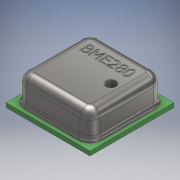
# Autodesk Inventor part: 66-0007
Saved by Autodesk Inventor 2018 (Build 220112000, 112)
## iProperties
Created: 2020-01-30
Part Number: 66-0007
Material: Stainless Steel
Document SubType Name: Modeling
Designer: Bradley
Density: 8 g/cm^3
Appearance: Semi-Polished
Author: Bradley
Autodesk Inventor part; units mm, degrees
ref_plane "YZ Plane" through (0, 0, 0) normal (1, 0, 0) x (0, 1, 0)
ref_plane "XZ Plane" through (0, 0, 0) normal (0, 1, 0) x (-1, 0, 0)
ref_plane "XY Plane" through (0, 0, 0) normal (0, 0, 1) x (1, 0, 0)
sketch "Sketch1" plane through (0, 0, 0) normal (0, 0, 1) x (1, 0, 0)
  line L0 (-1.25, 1.25) -> (1.25, 1.25)
  line L1 (1.25, 1.25) -> (1.25, -1.25)
  line L2 (1.25, -1.25) -> (-1.25, -1.25)
  line L3 (-1.25, -1.25) -> (-1.25, 1.25)
  line L4 (-1.25, 1.25) -> (1.25, -1.25) construction
  line L5 (1.25, 1.25) -> (-1.25, -1.25) construction
  point P0 (0, 0)
  dimension "d0" = 2.5
  constraints: 12 end point, 2 midpoint, 2 parallel, 2 perpendicular, 1 horizontal
  measures "d0" distance of L1.end L2.end
extrude "Extrusion1" add sketch "Sketch1" along normal mid plane 0.13
sketch "Sketch2" plane through (0, 0, 0.065) normal (0, 0, 1) x (1, 0, 0)
  line L0 (1.25, 1.25) -> (-1.25, 1.25) projected
  line L1 (-1.25, 1.25) -> (-1.25, -1.25) projected
  line L2 (-1.25, -1.25) -> (1.25, -1.25) projected
  line L3 (1.25, -1.25) -> (1.25, 1.25) projected
  line L4 (-1.1, 1.1) -> (1.1, 1.1)
  line L5 (1.1, 1.1) -> (1.1, -1.1)
  line L6 (1.1, -1.1) -> (-1.1, -1.1)
  line L7 (-1.1, -1.1) -> (-1.1, 1.1)
  point P0 (0, 0)
  dimension "d3" = 2.2
  constraints: 8 end point, 3 other
  measures "d3" distance of L4.start L4.end
extrude "Extrusion2" add sketch "Sketch2" along normal blind 0.8 contours L4 L5 L6 L7
fillet "Fillet1" radius 0.3 4 edges at (1.1, 1.1, 0.465) (-1.1, 1.1, 0.465) (-1.1, -1.1, 0.465) (1.1, -1.1, 0.465)
fillet "Fillet1" radius 0.25 4 edges at (0, 1.1, 0.865) (-1.1, 0, 0.865) (1.1, 0, 0.865) (0, -1.1, 0.865)
fillet "Fillet1" radius 0.15 4 edges at (0, -1.1, 0.065) (1.1, 0, 0.065) (0, 1.1, 0.065) (-1.1, 0, 0.065)
sketch "Sketch3" plane through (0, 0, 0.865) normal (0, 0, 1) x (1, 0, 0)
  arc A0 (0.85, 0.8) -> (0.8, 0.85) centre (0.8, 0.8) ccw projected
  line L0 (-0.8, 0.85) -> (0.8, 0.85) projected
  arc A1 (-0.8, 0.85) -> (-0.85, 0.8) centre (-0.8, 0.8) ccw projected
  line L1 (-0.85, -0.8) -> (-0.85, 0.8) projected
  arc A2 (-0.85, -0.8) -> (-0.8, -0.85) centre (-0.8, -0.8) ccw projected
  line L2 (0.8, -0.85) -> (-0.8, -0.85) projected
  arc A3 (0.8, -0.85) -> (0.85, -0.8) centre (0.8, -0.8) ccw projected
  line L3 (0.85, 0.8) -> (0.85, -0.8) projected
  arc A4 (1.15, 0.8) -> (0.8, 1.15) centre (0.8, 0.8) ccw
  line L4 (1.15, 0.8) -> (1.15, -0.8)
  arc A5 (0.8, -1.15) -> (1.15, -0.8) centre (0.8, -0.8) ccw
  line L5 (0.8, -1.15) -> (-0.8, -1.15)
  arc A6 (-1.15, -0.8) -> (-0.8, -1.15) centre (-0.8, -0.8) ccw
  line L6 (-1.15, -0.8) -> (-1.15, 0.8)
  arc A7 (-0.8, 1.15) -> (-1.15, 0.8) centre (-0.8, 0.8) ccw
  line L7 (-0.8, 1.15) -> (0.8, 1.15)
  line L8 (-1.25, 1.25) -> (1.25, 1.25) projected
  line L9 (1.25, 1.25) -> (1.25, -1.25) projected
  line L10 (1.25, -1.25) -> (-1.25, -1.25) projected
  line L11 (-1.25, -1.25) -> (-1.25, 1.25) projected
  point P0 (0, 0)
  dimension "d9" = 2.3
  constraints: 8 end point, 8 point on circle, 4 centre point, 7 other
  measures "d9" distance between parallel lines of L4 L6
extrude "Extrusion3" cut sketch "Sketch3" against normal up to surface (0.8 mm away) contours L8 L9 L10 L11
sketch "Sketch4" plane through (0, 0, 0.865) normal (0, 0, 1) x (1, 0, 0)
  circle A0 centre (0.625, 0) radius 0.15
  line L0 (1.25, -1.25) -> (1.25, 1.25) projected
  point P0 (0, 0)
  dimension "d12" = 0.3
  dimension "d13" = 0.625
  constraints: 1 centre point, 1 horizontal alignment
  measures "d12" diameter of A0
  measures "d13" distance from line of L0 A0.centre
extrude "Extrusion4" cut sketch "Sketch4" against normal blind 0.8
sketch "Sketch5" plane through (0, 0, -0.065) normal (0, 0, -1) x (-1, 0, 0)
  line L0 (1.25, 1.25) -> (-1.25, 1.25) projected
  line L1 (-1.25, 1.25) -> (-1.25, -1.25) projected
  line L2 (-1.25, -1.25) -> (1.25, -1.25) projected
  line L3 (1.25, -1.25) -> (1.25, 1.25) projected
  line L4 (1.15, 1.15) -> (0.8, 1.15)
  line L5 (0.8, 1.15) -> (0.8, 0.8)
  line L6 (0.8, 0.8) -> (1.15, 0.8)
  line L7 (1.15, 0.8) -> (1.15, 1.15)
  line L8 (-1.15, 1.15) -> (-1.15, 0.8)
  line L9 (-1.15, 0.8) -> (-0.8, 0.8)
  line L10 (-0.8, 0.8) -> (-0.8, 1.15)
  line L11 (-0.8, 1.15) -> (-1.15, 1.15)
  line L12 (0.8, 0.5) -> (0.8, 0.15)
  line L13 (0.8, 0.15) -> (1.15, 0.15)
  line L14 (1.15, 0.15) -> (1.15, 0.5)
  line L15 (1.15, 0.5) -> (0.8, 0.5)
  line L16 (-1.15, 0.5) -> (-1.15, 0.15)
  line L17 (-1.15, 0.15) -> (-0.8, 0.15)
  line L18 (-0.8, 0.15) -> (-0.8, 0.5)
  line L19 (-0.8, 0.5) -> (-1.15, 0.5)
  line L20 (0.8, -0.15) -> (0.8, -0.5)
  line L21 (0.8, -0.5) -> (1.15, -0.5)
  line L22 (1.15, -0.5) -> (1.15, -0.15)
  line L23 (1.15, -0.15) -> (0.8, -0.15)
  line L24 (-1.15, -0.15) -> (-1.15, -0.5)
  line L25 (-1.15, -0.5) -> (-0.8, -0.5)
  line L26 (-0.8, -0.5) -> (-0.8, -0.15)
  line L27 (-0.8, -0.15) -> (-1.15, -0.15)
  line L28 (0.8, -0.8) -> (0.8, -1.15)
  line L29 (0.8, -1.15) -> (1.15, -1.15)
  line L30 (1.15, -1.15) -> (1.15, -0.8)
  line L31 (1.15, -0.8) -> (0.8, -0.8)
  line L32 (-1.15, -0.8) -> (-1.15, -1.15)
  line L33 (-1.15, -1.15) -> (-0.8, -1.15)
  line L34 (-0.8, -1.15) -> (-0.8, -0.8)
  line L35 (-0.8, -0.8) -> (-1.15, -0.8)
  circle A0 centre (-0.5, -0.975) radius 0.1
  point P0 (0, 0)
  point P1 (-0.8, -0.975)
  dimension "d16" = 0.35
  dimension "d19" = 1.95
  dimension "d22" = 0.65
  dimension "d25" = 0.75
  dimension "d26" = 0.1
  dimension "d27" = 0.1
  dimension "d28" = 0.2
  constraints: 64 end point, 2 horizontal, 2 parallel, 2 perpendicular, 1 centre point, 1 horizontal alignment, 1 midpoint, 1 vertical, 56 other
  measures "d16" distance of L6.end L5.end
  measures "d19" distance of L4.end L8.start
  measures "d22" distance of L4.end L12.start
  measures "d25" distance from line of A0.centre L1
  measures "d26" distance between parallel lines of L2 L29
  measures "d27" distance between parallel lines of L3 L30
  measures "d28" diameter of A0
extrude "Extrusion5" add sketch "Sketch5" along normal blind 0.02 contours L7 L6 L5 L4 | L11 L10 L9 L8 | L15 L14 L13 L12 | L19 L18 L17 L16 | L23 L22 L21 L20 | L27 L26 L25 L24 | L31 L30 L29 L28 | L35 L34 L33 L32 | A0
sketch "Sketch6" plane through (0, 0, 0.865) normal (0, 0, 1) x (1, 0, 0)
  circle A0 centre (0.625, 0) radius 0.15 construction
  arc A1 (0.85, 0.8) -> (0.8, 0.85) centre (0.8, 0.8) ccw construction
  line L0 (-0.8, 0.85) -> (0.8, 0.85) construction
  arc A2 (-0.8, 0.85) -> (-0.85, 0.8) centre (-0.8, 0.8) ccw construction
  line L1 (-0.85, -0.8) -> (-0.85, 0.8) construction
  arc A3 (-0.85, -0.8) -> (-0.8, -0.85) centre (-0.8, -0.8) ccw construction
  line L2 (0.8, -0.85) -> (-0.8, -0.85) construction
  arc A4 (0.8, -0.85) -> (0.85, -0.8) centre (0.8, -0.8) ccw construction
  line L3 (0.85, 0.8) -> (0.85, -0.8) construction
  line L4 (-0.85, 0.4) -> (0.8354, 0.4) construction
  spline S0 degree 2 poles (-0.5074, 0.4921) (-0.5074, 0.4698) (-0.5244, 0.4355) (-0.5385, 0.4243) knots 0 0 0 1 2 2 2
  spline S1 degree 2 poles (-0.5385, 0.4243) (-0.5555, 0.4112) (-0.5942, 0.4) (-0.6248, 0.4) knots 0 0 0 1 2 2 2
  line L5 (-0.6248, 0.4) -> (-0.7109, 0.4)
  line L6 (-0.7109, 0.4) -> (-0.7109, 0.7)
  line L7 (-0.7109, 0.7) -> (-0.6314, 0.7)
  spline S2 degree 2 poles (-0.6314, 0.7) (-0.5993, 0.7) (-0.5672, 0.6959) (-0.5526, 0.6878) knots 0 0 0 1 2 2 2
  spline S3 degree 2 poles (-0.5526, 0.6878) (-0.5363, 0.6793) (-0.5215, 0.6514) (-0.5215, 0.6324) knots 0 0 0 1 2 2 2
  spline S4 degree 2 poles (-0.5215, 0.6324) (-0.5215, 0.6113) (-0.5439, 0.5777) (-0.5636, 0.5682) knots 0 0 0 1 2 2 2
  line L8 (-0.5636, 0.5682) -> (-0.5636, 0.5668)
  spline S5 degree 2 poles (-0.5636, 0.5668) (-0.5368, 0.5595) (-0.5074, 0.5208) (-0.5074, 0.4921) knots 0 0 0 1 2 2 2
  spline S6 degree 2 poles (-0.549, 0.4904) (-0.549, 0.5075) (-0.5587, 0.5293) (-0.5733, 0.5371) knots 0 0 0 1 2 2 2
  spline S7 degree 2 poles (-0.5733, 0.5371) (-0.5828, 0.542) (-0.6051, 0.5449) (-0.6258, 0.5449) knots 0 0 0 1 2 2 2
  line L9 (-0.6258, 0.5449) -> (-0.671, 0.5449)
  line L10 (-0.671, 0.5449) -> (-0.671, 0.434)
  line L11 (-0.671, 0.434) -> (-0.6387, 0.434)
  spline S8 degree 2 poles (-0.6387, 0.434) (-0.6124, 0.434) (-0.5823, 0.4389) (-0.5706, 0.4467) knots 0 0 0 1 2 2 2
  spline S9 degree 2 poles (-0.5706, 0.4467) (-0.5594, 0.4547) (-0.549, 0.4746) (-0.549, 0.4904) knots 0 0 0 1 2 2 2
  spline S10 degree 2 poles (-0.5631, 0.6268) (-0.5631, 0.6375) (-0.5704, 0.6536) (-0.5784, 0.6582) knots 0 0 0 1 2 2 2
  spline S11 degree 2 poles (-0.5784, 0.6582) (-0.5881, 0.6635) (-0.6117, 0.666) (-0.6328, 0.666) knots 0 0 0 1 2 2 2
  line L12 (-0.6328, 0.666) -> (-0.671, 0.666)
  line L13 (-0.671, 0.666) -> (-0.671, 0.5782)
  line L14 (-0.671, 0.5782) -> (-0.6258, 0.5782)
  spline S12 degree 2 poles (-0.6258, 0.5782) (-0.6071, 0.5782) (-0.5893, 0.5821) (-0.5799, 0.5882) knots 0 0 0 1 2 2 2
  spline S13 degree 2 poles (-0.5799, 0.5882) (-0.5706, 0.594) (-0.5631, 0.6127) (-0.5631, 0.6268) knots 0 0 0 1 2 2 2
  line L15 (-0.2106, 0.4) -> (-0.2504, 0.4)
  line L16 (-0.2504, 0.4) -> (-0.2504, 0.6584)
  line L17 (-0.2504, 0.6584) -> (-0.3287, 0.4827)
  line L18 (-0.3287, 0.4827) -> (-0.353, 0.4827)
  line L19 (-0.353, 0.4827) -> (-0.4306, 0.6584)
  line L20 (-0.4306, 0.6584) -> (-0.4306, 0.4)
  line L21 (-0.4306, 0.4) -> (-0.4678, 0.4)
  line L22 (-0.4678, 0.4) -> (-0.4678, 0.7)
  line L23 (-0.4678, 0.7) -> (-0.4133, 0.7)
  line L24 (-0.4133, 0.7) -> (-0.3384, 0.533)
  line L25 (-0.3384, 0.533) -> (-0.266, 0.7)
  line L26 (-0.266, 0.7) -> (-0.2106, 0.7)
  line L27 (-0.2106, 0.7) -> (-0.2106, 0.4)
  line L28 (-0.1498, 0.4) -> (-0.1498, 0.7)
  line L29 (-0.1498, 0.7) -> (0.0379, 0.7)
  line L30 (0.0379, 0.7) -> (0.0379, 0.6645)
  line L31 (0.0379, 0.6645) -> (-0.1099, 0.6645)
  line L32 (-0.1099, 0.6645) -> (-0.1099, 0.5823)
  line L33 (-0.1099, 0.5823) -> (0.0279, 0.5823)
  line L34 (0.0279, 0.5823) -> (0.0279, 0.5468)
  line L35 (0.0279, 0.5468) -> (-0.1099, 0.5468)
  line L36 (-0.1099, 0.5468) -> (-0.1099, 0.4355)
  line L37 (-0.1099, 0.4355) -> (0.0379, 0.4355)
  line L38 (0.0379, 0.4355) -> (0.0379, 0.4)
  line L39 (0.0379, 0.4) -> (-0.1498, 0.4)
  line L40 (0.2582, 0.4) -> (0.0731, 0.4)
  line L41 (0.0731, 0.4) -> (0.0731, 0.4425)
  spline S14 degree 2 poles (0.0731, 0.4425) (0.0931, 0.4613) (0.1286, 0.496) (0.1456, 0.5147) knots 0 0 0 1 2 2 2
  spline S15 degree 2 poles (0.1456, 0.5147) (0.1799, 0.5524) (0.2049, 0.5976) (0.2049, 0.6217) knots 0 0 0 1 2 2 2
  spline S16 degree 2 poles (0.2049, 0.6217) (0.2049, 0.6344) (0.1971, 0.6533) (0.1901, 0.6594) knots 0 0 0 1 2 2 2
  spline S17 degree 2 poles (0.1901, 0.6594) (0.183, 0.6655) (0.1646, 0.6716) (0.1534, 0.6716) knots 0 0 0 1 2 2 2
  spline S18 degree 2 poles (0.1534, 0.6716) (0.1427, 0.6716) (0.1208, 0.6662) (0.1108, 0.6621) knots 0 0 0 1 2 2 2
  spline S19 degree 2 poles (0.1108, 0.6621) (0.1023, 0.6587) (0.0865, 0.6489) (0.0817, 0.6455) knots 0 0 0 1 2 2 2
  line L42 (0.0817, 0.6455) -> (0.0795, 0.6455)
  line L43 (0.0795, 0.6455) -> (0.0795, 0.6883)
  spline S20 degree 2 poles (0.0795, 0.6883) (0.0919, 0.6944) (0.1364, 0.7063) (0.1563, 0.7063) knots 0 0 0 1 2 2 2
  spline S21 degree 2 poles (0.1563, 0.7063) (0.1984, 0.7063) (0.2458, 0.6618) (0.2458, 0.6239) knots 0 0 0 1 2 2 2
  spline S22 degree 2 poles (0.2458, 0.6239) (0.2458, 0.6062) (0.2375, 0.5765) (0.2302, 0.5639) knots 0 0 0 1 2 2 2
  spline S23 degree 2 poles (0.2302, 0.5639) (0.2229, 0.5507) (0.2018, 0.525) (0.1901, 0.5126) knots 0 0 0 1 2 2 2
  spline S24 degree 2 poles (0.1901, 0.5126) (0.1711, 0.4919) (0.1247, 0.4476) (0.1108, 0.4348) knots 0 0 0 1 2 2 2
  line L44 (0.1108, 0.4348) -> (0.2582, 0.4348)
  line L45 (0.2582, 0.4348) -> (0.2582, 0.4)
  spline S25 degree 2 poles (0.3889, 0.3932) (0.3666, 0.3932) (0.3299, 0.4066) (0.317, 0.419) knots 0 0 0 1 2 2 2
  spline S26 degree 2 poles (0.317, 0.419) (0.3043, 0.4311) (0.2912, 0.4642) (0.2912, 0.4829) knots 0 0 0 1 2 2 2
  spline S27 degree 2 poles (0.2912, 0.4829) (0.2912, 0.5072) (0.3172, 0.5481) (0.342, 0.5602) knots 0 0 0 1 2 2 2
  line L46 (0.342, 0.5602) -> (0.342, 0.5614)
  spline S28 degree 2 poles (0.342, 0.5614) (0.3199, 0.5743) (0.2985, 0.6049) (0.2985, 0.6278) knots 0 0 0 1 2 2 2
  spline S29 degree 2 poles (0.2985, 0.6278) (0.2985, 0.6616) (0.3496, 0.7068) (0.3889, 0.7068) knots 0 0 0 1 2 2 2
  spline S30 degree 2 poles (0.3889, 0.7068) (0.4298, 0.7068) (0.4791, 0.664) (0.4791, 0.6305) knots 0 0 0 1 2 2 2
  spline S31 degree 2 poles (0.4791, 0.6305) (0.4791, 0.6103) (0.4556, 0.5709) (0.4334, 0.5597) knots 0 0 0 1 2 2 2
  line L47 (0.4334, 0.5597) -> (0.4334, 0.5585)
  spline S32 degree 2 poles (0.4334, 0.5585) (0.4597, 0.5464) (0.4867, 0.5113) (0.4867, 0.4836) knots 0 0 0 1 2 2 2
  spline S33 degree 2 poles (0.4867, 0.4836) (0.4867, 0.4452) (0.4308, 0.3932) (0.3889, 0.3932) knots 0 0 0 1 2 2 2
  spline S34 degree 2 poles (0.4454, 0.4797) (0.4454, 0.4982) (0.4308, 0.5201) (0.4101, 0.5313) knots 0 0 0 1 2 2 2
  spline S35 degree 2 poles (0.4101, 0.5313) (0.4033, 0.5352) (0.3804, 0.5442) (0.3661, 0.55) knots 0 0 0 1 2 2 2
  spline S36 degree 2 poles (0.3661, 0.55) (0.3496, 0.5391) (0.3318, 0.5065) (0.3318, 0.4858) knots 0 0 0 1 2 2 2
  spline S37 degree 2 poles (0.3318, 0.4858) (0.3318, 0.4586) (0.3646, 0.4231) (0.3894, 0.4231) knots 0 0 0 1 2 2 2
  spline S38 degree 2 poles (0.3894, 0.4231) (0.4147, 0.4231) (0.4454, 0.4535) (0.4454, 0.4797) knots 0 0 0 1 2 2 2
  spline S39 degree 2 poles (0.4398, 0.63) (0.4398, 0.6502) (0.4128, 0.6771) (0.3887, 0.6771) knots 0 0 0 1 2 2 2
  spline S40 degree 2 poles (0.3887, 0.6771) (0.3668, 0.6771) (0.3389, 0.6531) (0.3389, 0.6324) knots 0 0 0 1 2 2 2
  spline S41 degree 2 poles (0.3389, 0.6324) (0.3389, 0.6176) (0.3532, 0.5969) (0.3676, 0.5887) knots 0 0 0 1 2 2 2
  spline S42 degree 2 poles (0.3676, 0.5887) (0.3736, 0.5853) (0.3994, 0.5733) (0.4099, 0.5699) knots 0 0 0 1 2 2 2
  spline S43 degree 2 poles (0.4099, 0.5699) (0.4274, 0.5833) (0.4398, 0.6118) (0.4398, 0.63) knots 0 0 0 1 2 2 2
  spline S44 degree 2 poles (0.7101, 0.55) (0.7101, 0.4693) (0.6632, 0.3937) (0.6143, 0.3937) knots 0 0 0 1 2 2 2
  spline S45 degree 2 poles (0.6143, 0.3937) (0.5647, 0.3937) (0.5183, 0.4707) (0.5183, 0.5498) knots 0 0 0 1 2 2 2
  spline S46 degree 2 poles (0.5183, 0.5498) (0.5183, 0.631) (0.5652, 0.7061) (0.6143, 0.7061) knots 0 0 0 1 2 2 2
  spline S47 degree 2 poles (0.6143, 0.7061) (0.6637, 0.7061) (0.7101, 0.6283) (0.7101, 0.55) knots 0 0 0 1 2 2 2
  spline S48 degree 2 poles (0.6586, 0.4586) (0.6644, 0.4734) (0.6693, 0.5191) (0.6693, 0.55) knots 0 0 0 1 2 2 2
  spline S49 degree 2 poles (0.6693, 0.55) (0.6693, 0.5809) (0.6644, 0.6263) (0.6583, 0.6417) knots 0 0 0 1 2 2 2
  spline S50 degree 2 poles (0.6583, 0.6417) (0.6522, 0.657) (0.6311, 0.6728) (0.6143, 0.6728) knots 0 0 0 1 2 2 2
  spline S51 degree 2 poles (0.6143, 0.6728) (0.5975, 0.6728) (0.5759, 0.657) (0.5696, 0.6412) knots 0 0 0 1 2 2 2
  spline S52 degree 2 poles (0.5696, 0.6412) (0.5635, 0.6259) (0.5591, 0.5792) (0.5591, 0.5498) knots 0 0 0 1 2 2 2
  spline S53 degree 2 poles (0.5591, 0.5498) (0.5591, 0.5182) (0.563, 0.4759) (0.5693, 0.4593) knots 0 0 0 1 2 2 2
  spline S54 degree 2 poles (0.5693, 0.4593) (0.5752, 0.4438) (0.5968, 0.427) (0.6143, 0.427) knots 0 0 0 1 2 2 2
  spline S55 degree 2 poles (0.6143, 0.427) (0.6308, 0.427) (0.6525, 0.4428) (0.6586, 0.4586) knots 0 0 0 1 2 2 2
  point P0 (0, 0)
  dimension "d31" = 0.4
  constraints: 2 end point, 2 horizontal, 1 point on line
  measures "d31" distance from line of point (0, 0) L4
extrude "Extrusion6" cut sketch "Sketch6" against normal blind 0.01
equation "\"d27\" = d26"
body "Solid1"
